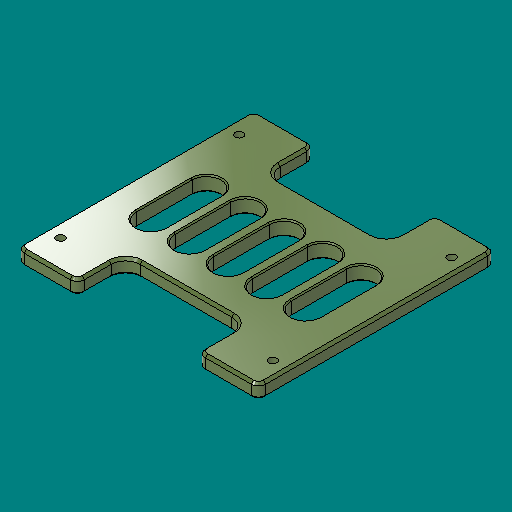
# Autodesk Inventor part: Cover-Plate-short-with-holes
Saved by Autodesk Inventor 2025 (Build 290162000, 162)
## iProperties
Created: 2023-12-01
Part Number: Cover-Plate-short-with-holes
Material: Generic
Document SubType Name: Modeling
Designer: kuzmin
Density: 1 g/cm^3
Appearance: Dark Olive
Author: kuzmin
Autodesk Inventor part; units mm, degrees
ref_plane "YZ Plane" through (0, 0, 0) normal (1, 0, 0) x (0, 1, 0)
ref_plane "XZ Plane" through (0, 0, 0) normal (0, 1, 0) x (-1, 0, 0)
ref_plane "XY Plane" through (0, 0, 0) normal (0, 0, 1) x (1, 0, 0)
sketch "Sketch1" plane through (0, 0, 0) normal (0, 0, 1) x (1, 0, 0)
  line L0 (-49, 50) -> (49, 50)
  line L1 (49, 50) -> (49, -50)
  line L2 (49, -50) -> (-49, -50)
  line L3 (-49, -50) -> (-49, 50)
  point P0 (0, 0)
  point P1 (0, 50)
  point P2 (49, 0)
  dimension "d2" = 100
  dimension "d3" = 98
  constraints: 8 end point, 2 midpoint, 2 parallel, 1 horizontal, 1 horizontal alignment, 1 perpendicular, 1 vertical alignment
  measures "d2" distance of L0.end L1.end
  measures "d3" distance of L0.start L0.end
extrude "Extrusion1" add sketch "Sketch1" along normal blind 6
sketch "Sketch5" plane through (0, 0, 6) normal (0, 0, 1) x (1, 0, 0)
  circle A0 centre (37, -43.9615) radius 1.7
  circle A1 centre (37, 43.9615) radius 1.7
  line L0 (37, -43.9615) -> (37, 43.9615) construction
  line L1 (49, -50) -> (49, 50) projected
  point P0 (0, 0)
  point P1 (37, 0)
  point P2 (49, 0)
  dimension "d27" = 3.4
  dimension "d28" = 12
  dimension "d29" = 87.923
  constraints: 2 centre point, 2 end point, 2 midpoint, 1 equal radius, 1 horizontal alignment, 1 vertical
  measures "d27" diameter of A0
  measures "d28" distance between parallel lines of L1 L0
  measures "d29" distance of L0.start L0.end
extrude "Extrusion5" cut sketch "Sketch5" against normal through all
sketch "Sketch6" plane through (0, 0, 6) normal (0, 0, 1) x (1, 0, 0)
  line L0 (29, 25) -> (49, 25)
  line L1 (49, 25) -> (49, -25)
  line L2 (49, -25) -> (29, -25)
  line L3 (29, -25) -> (29, 25)
  line L4 (49, -50) -> (49, 50) projected
  point P0 (0, 0)
  point P1 (49, 0)
  dimension "d34" = 20
  dimension "d35" = 50
  constraints: 8 end point, 2 midpoint, 2 parallel, 1 horizontal, 1 perpendicular
  measures "d34" distance of L0.start L0.end
  measures "d35" distance of L2.end L0.start
extrude "Extrusion6" cut sketch "Sketch6" against normal through all
fillet "Fillet2" radius 6 2 edges at (29, -25, 3) (29, 25, 3)
fillet "Fillet3" radius 3 6 edges at (49, -25, 3) (49, -50, 3) (49, 25, 3) (49, 50, 3) (-49, 50, 3) (-49, -50, 3)
mirror "Mirror1" about plane through (0, 0, 0) normal (1, 0, 0) of "Extrusion5", "Extrusion6", "Fillet2", "Fillet3"
chamfer "Chamfer5" distance 1 angle 45 34 edges at (0, -50, 6) (48.1213, -49.1213, 6) (49, -37.5, 6) (48.1213, -25.8787, 6) (40.5, -25, 6) (30.7574, -23.2426, 6) (29, 0, 6) (30.7574, 23.2426, 6) (40.5, 25, 6) (48.1213, 25.8787, 6) (49, 37.5, 6) (48.1213, 49.1213, 6) (0, 50, 6) (-48.1213, 49.1213, 6) (-49, 37.5, 6) (-49, -37.5, 6) (-48.1213, -49.1213, 6) (0, 50, 0) (-48.1213, 49.1213, 0) (-49, 37.5, 0) (-49, -37.5, 0) (-48.1213, -49.1213, 0) (0, -50, 0) (48.1213, -49.1213, 0) (49, -37.5, 0) (48.1213, -25.8787, 0) (40.5, -25, 0) (30.7574, -23.2426, 0) (29, 0, 0) (30.7574, 23.2426, 0) (40.5, 25, 0) (48.1213, 25.8787, 0) (49, 37.5, 0) (48.1213, 49.1213, 0)
sketch "Sketch11" plane through (0, 0, 6) normal (0, 0, 1) x (1, 0, 0)
  line L0 (17.5, -6) -> (-17.5, -6)
  line L1 (-17.5, -6) -> (-17.5, 6)
  line L2 (-17.5, 6) -> (17.5, 6)
  line L3 (17.5, 6) -> (17.5, -6)
  point P0 (0, 0)
  point P1 (-17.5, 0)
  point P2 (0, -6)
  dimension "d60" = 35
  dimension "d61" = 12
  constraints: 8 end point, 2 midpoint, 2 parallel, 1 horizontal, 1 horizontal alignment, 1 perpendicular, 1 vertical alignment
  measures "d60" distance of L0.start L0.end
  measures "d61" distance of L0.end L1.end
extrude "Extrusion10" cut sketch "Sketch11" against normal through all
fillet "Fillet5" radius 6 4 edges at (17.5, -6, 3) (-17.5, -6, 3) (-17.5, 6, 3) (17.5, 6, 3)
chamfer "Chamfer6" distance 0.5 angle 45 8 edges at (0, -6, 6) (-15.7427, -4.2427, 6) (0, 6, 6) (15.7427, -4.2427, 6) (0, -6, 0) (15.7427, -4.2427, 0) (0, 6, 0) (-15.7427, -4.2427, 0)
pattern_linear "Rectangular Pattern1" count 5 spacing 16 along (0, 1, 0) of "Extrusion10", "Fillet5", "Chamfer6" first direction both ways yes
body "Solid1"
